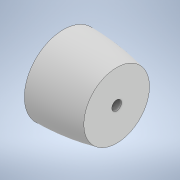
# Autodesk Inventor part: roller_half
Saved by Autodesk Inventor 2021 (Build 250183000, 183)
## iProperties
Created: 2022-10-17
Part Number: roller_half
Material: Generic
Document SubType Name: Modeling
Designer: Jonathan
Density: 1 g/cm^3
Appearance: Default
Author: Jonathan
Autodesk Inventor part; units mm, degrees
ref_plane "YZ Plane" through (0, 0, 0) normal (1, 0, 0) x (0, 1, 0)
ref_plane "XZ Plane" through (0, 0, 0) normal (0, 1, 0) x (-1, 0, 0)
ref_plane "XY Plane" through (0, 0, 0) normal (0, 0, 1) x (1, 0, 0)
sketch "Sketch1" plane through (0, 0, 0) normal (0, 1, 0) x (-1, 0, 0)
  line L0 (0, 0) -> (0, 47.7364) construction
  line L1 (0, 47.7364) -> (-17.3746, 0) construction
  line L2 (-17.3746, 0) -> (0, 0) construction
  line L3 (0, 0) -> (17.3746, 0) construction
  line L4 (0, 0) -> (0, -12.7) construction
  arc A0 (-17.3746, -10.6927) -> (17.3746, -10.6927) centre (0, 63.5) ccw construction
  line L5 (-17.3746, 0) -> (-17.3746, -10.6927) construction
  line L6 (17.3746, 0) -> (17.3746, -10.6927) construction
  line L7 (-17.3746, -10.6927) -> (-17.3746, -1.5875)
  line L8 (-17.3746, -1.5875) -> (0, -1.5875)
  line L9 (0, -12.7) -> (0, -1.5875)
  arc A1 (-17.3746, -10.6927) -> (0, -12.7) centre (0, 63.5) ccw
  dimension "d0" = 50.8
  dimension "d1" = 20
  dimension "d2" = 12.7
  dimension "d4" = 76.2
  dimension "d7" = 1.5875
  constraints: 20 end point, 5 point on circle, 4 vertical, 3 point on line, 2 centre point, 2 collinear, 2 equal length, 1 coincident, 1 concentric, 1 horizontal, 1 perpendicular
  measures "d0" distance of L0.end L1.end
  measures "d1" angle of L0 L1
  measures "d2" distance of L2.end L4.end
  measures "d4" distance of A0.centre L4.end
  measures "d7" distance between parallel lines of L8 L2
revolve "Revolution1" add sketch "Sketch1" angle 360 about axis through (0, 0, 0) along (1, 0, 0)
equation "\"d0\" = 0.5 * wheel_d - roller_d"
equation "\"d1\" = 0.5 * roller_angle"
equation "\"d2\" = 0.5 * roller_d"
equation "\"d4\" = 0.5 * wheel_d"
equation "\"d7\" = 0.5 * roller_shaft_d"
equation "\"wheel_d\" = 152.4"
equation "\"roller_d\" = 25.4"
equation "\"roller_angle\" = 40deg"
equation "\"roller_shaft_d\" = 3.175"
body "Solid1"
